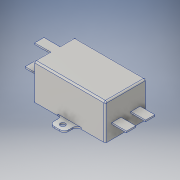
# Autodesk Inventor part: Netzfilter
Saved by Autodesk Inventor 2016 (Build 200138000, 138)
## iProperties
Created: 2018-05-16
Part Number: Netzfilter
Material: Aluminum 6061
Document SubType Name: Modeling
Designer: Phil Erle
Density: 2.7 g/cm^3
Appearance: Aluminum - Flat
Author: Phil Erle
Autodesk Inventor part; units mm, degrees
ref_plane "YZ Plane" through (0, 0, 0) normal (1, 0, 0) x (0, 1, 0)
ref_plane "XZ Plane" through (0, 0, 0) normal (0, 1, 0) x (-1, 0, 0)
ref_plane "XY Plane" through (0, 0, 0) normal (0, 0, 1) x (1, 0, 0)
sketch "Sketch1" plane through (0, 0, 0) normal (0, 0, 1) x (1, 0, 0)
  line L0 (-24.5, -14) -> (24.5, -14)
  line L1 (24.5, -14) -> (24.5, 14)
  line L2 (24.5, 14) -> (-24.5, 14)
  line L3 (-24.5, 14) -> (-24.5, -14)
  line L4 (-24.5, -14) -> (24.5, 14) construction
  line L5 (24.5, -14) -> (-24.5, 14) construction
  point P0 (0, 0)
  dimension "d0" = 49
  dimension "d1" = 28
  constraints: 12 end point, 2 midpoint, 2 parallel, 1 horizontal, 1 perpendicular
  measures "d0" distance of L1.end L2.end
  measures "d1" distance of L0.end L1.end
extrude "Extrusion1" add sketch "Sketch1" along normal blind 24.3
sketch "Sketch2" plane through (24.5, -14, 0) normal (1, 0, 0) x (0, 0, -1)
  line L0 (-9, 4.35) -> (-10, 4.35)
  line L1 (-10, 4.35) -> (-10, 10.65)
  line L2 (-10, 10.65) -> (-9, 10.65)
  line L3 (-9, 10.65) -> (-9, 4.35)
  line L4 (-9, 4.35) -> (-10, 10.65) construction
  line L5 (-10, 4.35) -> (-9, 10.65) construction
  line L6 (-9, 17.35) -> (-10, 17.35)
  line L7 (-10, 17.35) -> (-10, 23.65)
  line L8 (-10, 23.65) -> (-9, 23.65)
  line L9 (-9, 23.65) -> (-9, 17.35)
  line L10 (-9, 17.35) -> (-10, 23.65) construction
  line L11 (-10, 17.35) -> (-9, 23.65) construction
  line L12 (-9.5, 7.5) -> (-9.5, 20.5) construction
  line L13 (0, 0) -> (0, 28) construction
  point P0 (0, 14)
  point P1 (-9.5, 14)
  point P2 (0, 14)
  dimension "d4" = 1
  dimension "d5" = 6.3
  dimension "d6" = 6.3
  dimension "d7" = 13
  dimension "d8" = 9
  constraints: 26 end point, 6 midpoint, 5 parallel, 2 horizontal, 2 perpendicular, 1 horizontal alignment, 1 point on line
  measures "d4" distance of L7.end L8.end
  measures "d5" distance of L6.end L7.end
  measures "d6" distance of L0.end L1.end
  measures "d7" distance of L12.end L12.start
  measures "d8" distance between parallel lines of L13 L3
extrude "Extrusion2" add sketch "Sketch2" along normal blind 10
sketch "Sketch3" plane through (-24.5, -14, 0) normal (0, -1, 0) x (1, 0, 0)
  line L0 (19.5, 0) -> (29.5, 0)
  line L1 (29.5, 0) -> (29.5, 1)
  line L2 (29.5, 1) -> (19.5, 1)
  line L3 (19.5, 1) -> (19.5, 0)
  line L4 (0, 0) -> (49, 0) projected
  point P0 (24.5, 0)
  point P1 (24.5, 0)
  point P2 (24.5, 0)
  point P3 (24.5, 0)
  dimension "d11" = 1
  dimension "d12" = 10
  constraints: 8 end point, 3 midpoint, 2 parallel, 1 coincident, 1 horizontal, 1 horizontal alignment, 1 perpendicular
  measures "d11" distance of L0.end L1.end
  measures "d12" distance of L1.end L2.end
extrude "Extrusion3" add sketch "Sketch3" along normal blind 8.5
sketch "Sketch4" plane through (-24.5, 14, 0) normal (0, 1, 0) x (1, 0, 0)
  line L0 (29.5, -1) -> (29.5, 0) projected
  line L1 (29.5, 0) -> (19.5, 0)
  line L2 (19.5, 0) -> (19.5, -1)
  line L3 (19.5, -1) -> (29.5, -1)
  line L4 (29.5, -1) -> (29.5, 0)
  line L5 (49, 0) -> (0, 0) projected
  point P0 (24.5, 0)
  point P1 (24.5, -1)
  point P2 (24.5, 0)
  dimension "d15" = 1
  constraints: 8 end point, 2 midpoint, 2 parallel, 1 horizontal, 1 perpendicular, 1 vertical alignment
  measures "d15" distance of L1.end L2.end
extrude "Extrusion4" add sketch "Sketch4" along normal blind 8.5
sketch "Sketch5" plane through (-24.5, -14, 0) normal (-1, 0, 0) x (0, 0, 1)
  line L0 (12.5, 23.65) -> (13.5, 23.65)
  line L1 (13.5, 23.65) -> (13.5, 17.35)
  line L2 (13.5, 17.35) -> (12.5, 17.35)
  line L3 (12.5, 17.35) -> (12.5, 23.65)
  line L4 (12.5, 23.65) -> (13.5, 17.35) construction
  line L5 (13.5, 23.65) -> (12.5, 17.35) construction
  line L6 (12.5, 4.35) -> (13.5, 4.35)
  line L7 (13.5, 4.35) -> (13.5, 10.65)
  line L8 (13.5, 10.65) -> (12.5, 10.65)
  line L9 (12.5, 10.65) -> (12.5, 4.35)
  line L10 (12.5, 4.35) -> (13.5, 10.65) construction
  line L11 (13.5, 4.35) -> (12.5, 10.65) construction
  line L12 (13, 20.5) -> (13, 7.5) construction
  line L13 (0, 28) -> (0, 0) construction
  point P0 (0, 14)
  point P1 (13, 14)
  point P2 (0, 14)
  dimension "d18" = 1
  dimension "d19" = 6.3
  dimension "d20" = 6.3
  dimension "d21" = 13
  dimension "d22" = 13
  constraints: 26 end point, 6 midpoint, 4 parallel, 2 horizontal, 2 perpendicular, 1 horizontal alignment, 1 point on line, 1 vertical
  measures "d18" distance of L0.start L0.end
  measures "d19" distance of L0.end L1.end
  measures "d20" distance of L6.end L7.end
  measures "d21" distance of L12.start L12.end
  measures "d22" distance from line of L12 point (0, 14)
extrude "Extrusion5" add sketch "Sketch5" along normal blind 10
sketch "Sketch6" plane through (-24.5, -14, 0) normal (-1, 0, 0) x (0, 0, 1)
  line L0 (23.3, 17.15) -> (24.3, 17.15)
  line L1 (24.3, 17.15) -> (24.3, 10.85)
  line L2 (24.3, 10.85) -> (23.3, 10.85)
  line L3 (23.3, 10.85) -> (23.3, 17.15)
  line L4 (23.3, 17.15) -> (24.3, 10.85) construction
  line L5 (24.3, 17.15) -> (23.3, 10.85) construction
  line L6 (0, 28) -> (0, 0) projected
  point P0 (0, 14)
  point P1 (23.8, 14)
  point P2 (23.8, 14)
  point P3 (0, 14)
  point P4 (24.3, 28)
  dimension "d25" = 1
  dimension "d26" = 6.3
  constraints: 12 end point, 4 midpoint, 2 parallel, 1 horizontal, 1 horizontal alignment, 1 perpendicular, 1 vertical alignment
  measures "d25" distance of L0.start L0.end
  measures "d26" distance of L0.end L1.end
extrude "Extrusion6" add sketch "Sketch6" along normal blind 10
fillet "Fillet1" radius 1 9 edges at (0, -14, 24.3) (-24.5, -8.575, 24.3) (-24.5, 8.575, 24.3) (-24.5, 14, 12.15) (0, 14, 24.3) (-24.5, -14, 12.15) (24.5, -14, 12.15) (24.5, 0, 24.3) (24.5, 14, 12.15)
fillet "Fillet2" radius 3 8 edges at (5, -14, 0.5) (5, -22.5, 0.5) (-5, -22.5, 0.5) (-5, -14, 0.5) (-5, 14, 0.5) (-5, 22.5, 0.5) (5, 14, 0.5) (5, 22.5, 0.5)
sketch "Sketch7" plane through (0, 0, 0) normal (0, 0, -1) x (-1, 0, 0)
  line L0 (0, 18.5) -> (0, -18.5) construction
  point P0 (0, 0)
  point P1 (0, 0)
  dimension "d31" = 37
  constraints: 3 coincident, 2 end point, 1 midpoint, 1 vertical, 1 vertical alignment
  measures "d31" distance of L0.start L0.end
hole "Hole1" at (0, 18.5, 0) at (0, -18.5, 0) direction (0, 0, 1) diameter 3.4 depth 8 tip angle 118 clearance for "Countersunk Flat Head Screw DIN EN ISO 2009" size "M3" standard "DIN"
body "Solid1"
